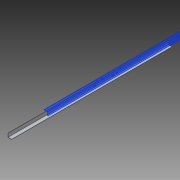
# Autodesk Inventor part: Shooter Back Support Bar
Saved by Autodesk Inventor 2014 SP1 (Build 180222100, 222)
## iProperties
Created: 2013-12-13
Part Number: Shooter Back Support Bar
Material: Aluminum 6061
Document SubType Name: Modeling
Designer: Moses
Mass: 45.3053 g
Surface Area: 433.276 cm^2
Volume: 16.7178 cm^3
Density: 2.71 g/cm^3
Appearance: Aluminum - Flat
Author: Moses
Autodesk Inventor part; units mm, degrees
ref_plane "YZ Plane" through (0, 0, 0) normal (1, 0, 0) x (0, 1, 0)
ref_plane "XZ Plane" through (0, 0, 0) normal (0, 1, 0) x (-1, 0, 0)
ref_plane "XY Plane" through (0, 0, 0) normal (0, 0, 1) x (1, 0, 0)
sketch "Sketch1" plane through (0, 0, 0) normal (0, 0, 1) x (1, 0, 0)
  line L0 (0, 0) -> (0, 15.875)
  line L1 (0, 15.875) -> (0.7937, 15.875)
  line L2 (0.7937, 15.875) -> (0.7938, 0.7937)
  line L3 (0.7938, 0.7937) -> (15.875, 0.7937)
  line L4 (15.875, 0.7937) -> (15.875, 0)
  line L5 (15.875, 0) -> (0, 0)
  dimension "d0" = 15.875
  dimension "d1" = 0.7937
  constraints: 12 end point, 3 horizontal, 3 vertical, 2 perpendicular
  measures "d0" distance of L0.start L0.end
  measures "d1" distance of L0.end L1.end
extrude "Extrusion1" add sketch "Sketch1" along normal blind 685.0063
sketch "Sketch2" plane through (0, 0, 0) normal (-1, 0, 0) x (0, 0, 1)
  line L0 (288.925, 278.403) -> (593.725, 278.403) construction
  arc A0 (593.725, 278.403) -> (593.725, 285.1594) centre (593.725, 281.7812) ccw construction
  line L1 (593.725, 285.1594) -> (288.925, 285.1594) construction
  arc A1 (288.925, 285.1594) -> (288.925, 278.403) centre (288.925, 281.7812) ccw construction
  circle A2 centre (657.225, 281.7812) radius 3.3782 construction
  circle A3 centre (625.475, 281.7812) radius 3.3782 construction
  line L2 (669.925, 294.4812) -> (669.925, 484.9812) construction
  line L3 (669.925, 484.9812) -> (200.025, 484.9812) construction
  line L4 (200.025, 484.9812) -> (200.025, 294.4812) construction
  line L5 (200.025, 294.4812) -> (669.925, 294.4812) construction
  line L6 (288.925, 151.403) -> (593.725, 151.403) construction
  arc A4 (593.725, 151.403) -> (593.725, 158.1594) centre (593.725, 154.7812) ccw construction
  line L7 (593.725, 158.1594) -> (288.925, 158.1594) construction
  arc A5 (288.925, 158.1594) -> (288.925, 151.403) centre (288.925, 154.7812) ccw construction
  ellipse E0 centre (657.225, 154.7796) end of major axis (653.8468, 154.7796) minor radius 3.3782 construction
  ellipse E1 centre (625.475, 154.7796) end of major axis (628.8532, 154.7796) minor radius 3.3782 construction
  line L8 (669.925, 269.0812) -> (200.025, 269.0812) construction
  line L9 (200.025, 269.0812) -> (200.025, 167.4812) construction
  line L10 (200.025, 167.4812) -> (669.925, 167.4812) construction
  line L11 (669.925, 167.4812) -> (669.925, 269.0812) construction
  line L12 (669.925, 15.0813) -> (669.925, 142.0812) construction
  line L13 (669.925, 142.0812) -> (200.025, 142.0812) construction
  line L14 (200.025, 142.0812) -> (200.025, 15.0813) construction
  line L15 (200.025, 15.0813) -> (669.925, 15.0813) construction
  circle A6 centre (676.275, 396.0812) radius 3.3782 construction
  circle A7 centre (193.675, 396.0812) radius 3.3782 construction
  circle A8 centre (676.275, 407.9875) radius 3.3782 construction
  circle A9 centre (193.675, 407.9875) radius 3.3782 construction
  circle A10 centre (676.275, 419.8937) radius 3.3782 construction
  circle A11 centre (193.675, 419.8937) radius 3.3782 construction
  circle A12 centre (676.275, 431.8) radius 3.3782 construction
  circle A13 centre (193.675, 431.8) radius 3.3782 construction
  circle A14 centre (676.275, 443.7062) radius 3.3782 construction
  circle A15 centre (193.675, 443.7062) radius 3.3782 construction
  circle A16 centre (676.275, 455.6125) radius 3.3782 construction
  circle A17 centre (193.675, 455.6125) radius 3.3782 construction
  circle A18 centre (676.275, 467.5187) radius 3.3782 construction
  circle A19 centre (193.675, 467.5187) radius 3.3782 construction
  circle A20 centre (676.275, 479.425) radius 3.3782 construction
  circle A21 centre (193.675, 479.425) radius 3.3782 construction
  circle A22 centre (676.275, 385.0141) radius 3.3782 construction
  circle A23 centre (193.675, 385.0141) radius 3.3782 construction
  circle A24 centre (676.275, 373.947) radius 3.3782 construction
  circle A25 centre (193.675, 373.947) radius 3.3782 construction
  circle A26 centre (676.275, 362.8798) radius 3.3782 construction
  circle A27 centre (193.675, 362.8798) radius 3.3782 construction
  circle A28 centre (676.275, 351.8127) radius 3.3782 construction
  circle A29 centre (193.675, 351.8127) radius 3.3782 construction
  circle A30 centre (676.275, 340.7455) radius 3.3782 construction
  circle A31 centre (193.675, 340.7455) radius 3.3782 construction
  circle A32 centre (676.275, 329.6784) radius 3.3782 construction
  circle A33 centre (193.675, 329.6784) radius 3.3782 construction
  circle A34 centre (676.275, 318.6112) radius 3.3782 construction
  circle A35 centre (193.675, 318.6112) radius 3.3782 construction
  circle A36 centre (676.275, 307.5441) radius 3.3782 construction
  circle A37 centre (193.675, 307.5441) radius 3.3782 construction
  circle A38 centre (676.275, 296.477) radius 3.3782 construction
  circle A39 centre (193.675, 296.477) radius 3.3782 construction
  circle A40 centre (676.275, 285.4098) radius 3.3782 construction
  circle A41 centre (193.675, 285.4098) radius 3.3782 construction
  circle A42 centre (676.275, 274.3427) radius 3.3782 construction
  circle A43 centre (193.675, 274.3427) radius 3.3782 construction
  circle A44 centre (676.275, 263.2755) radius 3.3782 construction
  circle A45 centre (193.675, 263.2755) radius 3.3782 construction
  circle A46 centre (676.275, 252.2084) radius 3.3782 construction
  circle A47 centre (193.675, 252.2084) radius 3.3782 construction
  circle A48 centre (676.275, 241.1412) radius 3.3782 construction
  circle A49 centre (193.675, 241.1412) radius 3.3782 construction
  circle A50 centre (676.275, 230.0741) radius 3.3782 construction
  circle A51 centre (193.675, 230.0741) radius 3.3782 construction
  circle A52 centre (676.275, 219.007) radius 3.3782 construction
  circle A53 centre (193.675, 219.007) radius 3.3782 construction
  circle A54 centre (676.275, 207.9398) radius 3.3782 construction
  circle A55 centre (193.675, 207.9398) radius 3.3782 construction
  circle A56 centre (676.275, 196.8727) radius 3.3782 construction
  circle A57 centre (193.675, 196.8727) radius 3.3782 construction
  circle A58 centre (676.275, 185.8055) radius 3.3782 construction
  circle A59 centre (193.675, 185.8055) radius 3.3782 construction
  circle A60 centre (676.275, 174.7384) radius 3.3782 construction
  circle A61 centre (193.675, 174.7384) radius 3.3782 construction
  circle A62 centre (676.275, 163.6712) radius 3.3782 construction
  circle A63 centre (193.675, 163.6712) radius 3.3782 construction
  circle A64 centre (676.275, 152.6041) radius 3.3782 construction
  circle A65 centre (193.675, 152.6041) radius 3.3782 construction
  circle A66 centre (676.275, 141.537) radius 3.3782 construction
  circle A67 centre (193.675, 141.537) radius 3.3782 construction
  circle A68 centre (676.275, 130.4698) radius 3.3782 construction
  circle A69 centre (193.675, 130.4698) radius 3.3782 construction
  circle A70 centre (676.275, 119.4027) radius 3.3782 construction
  circle A71 centre (193.675, 119.4027) radius 3.3782 construction
  circle A72 centre (676.275, 108.3355) radius 3.3782 construction
  circle A73 centre (193.675, 108.3355) radius 3.3782 construction
  circle A74 centre (676.275, 97.2684) radius 3.3782 construction
  circle A75 centre (193.675, 97.2684) radius 3.3782 construction
  circle A76 centre (676.275, 86.2012) radius 3.3782 construction
  circle A77 centre (193.675, 86.2012) radius 3.3782 construction
  circle A78 centre (676.275, 75.1341) radius 3.3782 construction
  circle A79 centre (193.675, 75.1341) radius 3.3782 construction
  circle A80 centre (676.275, 64.067) radius 3.3782 construction
  circle A81 centre (193.675, 64.067) radius 3.3782 construction
  circle A82 centre (676.275, 52.9998) radius 3.3782 construction
  circle A83 centre (193.675, 52.9998) radius 3.3782 construction
  circle A84 centre (676.275, 41.9327) radius 3.3782 construction
  circle A85 centre (193.675, 41.9327) radius 3.3782 construction
  circle A86 centre (676.275, 30.8655) radius 3.3782 construction
  circle A87 centre (193.675, 30.8655) radius 3.3782 construction
  circle A88 centre (676.275, 19.7984) radius 3.3782 construction
  circle A89 centre (193.675, 19.7984) radius 3.3782 construction
  circle A90 centre (676.275, 491.3312) radius 3.3782 construction
  circle A91 centre (666.426, 491.3312) radius 3.3782 construction
  circle A92 centre (656.577, 491.3312) radius 3.3782 construction
  circle A93 centre (646.7281, 491.3312) radius 3.3782 construction
  circle A94 centre (636.8791, 491.3312) radius 3.3782 construction
  circle A95 centre (627.0301, 491.3312) radius 3.3782 construction
  circle A96 centre (617.1811, 491.3312) radius 3.3782 construction
  circle A97 centre (607.3321, 491.3312) radius 3.3782 construction
  circle A98 centre (597.4832, 491.3312) radius 3.3782 construction
  circle A99 centre (587.6342, 491.3312) radius 3.3782 construction
  circle A100 centre (577.7852, 491.3312) radius 3.3782 construction
  circle A101 centre (567.9362, 491.3312) radius 3.3782 construction
  circle A102 centre (558.0872, 491.3312) radius 3.3782 construction
  circle A103 centre (548.2383, 491.3312) radius 3.3782 construction
  circle A104 centre (538.3893, 491.3312) radius 3.3782 construction
  circle A105 centre (528.5403, 491.3312) radius 3.3782 construction
  circle A106 centre (518.6913, 491.3312) radius 3.3782 construction
  circle A107 centre (508.8423, 491.3312) radius 3.3782 construction
  circle A108 centre (498.9934, 491.3312) radius 3.3782 construction
  circle A109 centre (489.1444, 491.3312) radius 3.3782 construction
  circle A110 centre (479.2954, 491.3312) radius 3.3782 construction
  circle A111 centre (469.4464, 491.3312) radius 3.3782 construction
  circle A112 centre (459.5974, 491.3312) radius 3.3782 construction
  circle A113 centre (449.7485, 491.3312) radius 3.3782 construction
  circle A114 centre (439.8995, 491.3312) radius 3.3782 construction
  circle A115 centre (430.0505, 491.3312) radius 3.3782 construction
  circle A116 centre (420.2015, 491.3312) radius 3.3782 construction
  circle A117 centre (410.3526, 491.3312) radius 3.3782 construction
  circle A118 centre (400.5036, 491.3312) radius 3.3782 construction
  circle A119 centre (390.6546, 491.3312) radius 3.3782 construction
  circle A120 centre (380.8056, 491.3312) radius 3.3782 construction
  circle A121 centre (370.9566, 491.3312) radius 3.3782 construction
  circle A122 centre (361.1077, 491.3312) radius 3.3782 construction
  circle A123 centre (351.2587, 491.3312) radius 3.3782 construction
  circle A124 centre (341.4097, 491.3312) radius 3.3782 construction
  circle A125 centre (331.5607, 491.3312) radius 3.3782 construction
  circle A126 centre (321.7117, 491.3312) radius 3.3782 construction
  circle A127 centre (311.8628, 491.3312) radius 3.3782 construction
  circle A128 centre (302.0138, 491.3312) radius 3.3782 construction
  circle A129 centre (292.1648, 491.3312) radius 3.3782 construction
  circle A130 centre (282.3158, 491.3312) radius 3.3782 construction
  circle A131 centre (272.4668, 491.3312) radius 3.3782 construction
  circle A132 centre (262.6179, 491.3312) radius 3.3782 construction
  circle A133 centre (252.7689, 491.3312) radius 3.3782 construction
  circle A134 centre (242.9199, 491.3312) radius 3.3782 construction
  circle A135 centre (233.0709, 491.3312) radius 3.3782 construction
  circle A136 centre (223.2219, 491.3312) radius 3.3782 construction
  circle A137 centre (213.373, 491.3312) radius 3.3782 construction
  circle A138 centre (203.524, 491.3312) radius 3.3782 construction
  circle A139 centre (193.675, 491.3312) radius 3.3782 construction
  circle A140 centre (676.275, 8.7313) radius 3.3782 projected
  circle A141 centre (666.426, 8.7313) radius 3.3782 construction
  circle A142 centre (656.577, 8.7313) radius 3.3782 construction
  circle A143 centre (646.7281, 8.7313) radius 3.3782 construction
  circle A144 centre (636.8791, 8.7313) radius 3.3782 construction
  circle A145 centre (627.0301, 8.7313) radius 3.3782 construction
  circle A146 centre (617.1811, 8.7313) radius 3.3782 construction
  circle A147 centre (607.3321, 8.7313) radius 3.3782 construction
  circle A148 centre (597.4832, 8.7313) radius 3.3782 construction
  circle A149 centre (587.6342, 8.7313) radius 3.3782 construction
  circle A150 centre (577.7852, 8.7313) radius 3.3782 construction
  circle A151 centre (567.9362, 8.7313) radius 3.3782 construction
  circle A152 centre (558.0872, 8.7313) radius 3.3782 construction
  circle A153 centre (548.2383, 8.7313) radius 3.3782 construction
  circle A154 centre (538.3893, 8.7313) radius 3.3782 construction
  circle A155 centre (528.5403, 8.7313) radius 3.3782 construction
  circle A156 centre (518.6913, 8.7313) radius 3.3782 construction
  circle A157 centre (508.8423, 8.7313) radius 3.3782 construction
  circle A158 centre (498.9934, 8.7313) radius 3.3782 construction
  circle A159 centre (489.1444, 8.7313) radius 3.3782 construction
  circle A160 centre (479.2954, 8.7313) radius 3.3782 construction
  circle A161 centre (469.4464, 8.7313) radius 3.3782 construction
  circle A162 centre (459.5974, 8.7313) radius 3.3782 construction
  circle A163 centre (449.7485, 8.7313) radius 3.3782 construction
  circle A164 centre (439.8995, 8.7313) radius 3.3782 construction
  circle A165 centre (430.0505, 8.7313) radius 3.3782 construction
  circle A166 centre (420.2015, 8.7313) radius 3.3782 construction
  circle A167 centre (410.3526, 8.7313) radius 3.3782 construction
  circle A168 centre (400.5036, 8.7313) radius 3.3782 construction
  circle A169 centre (390.6546, 8.7313) radius 3.3782 construction
  circle A170 centre (380.8056, 8.7313) radius 3.3782 construction
  circle A171 centre (370.9566, 8.7313) radius 3.3782 construction
  circle A172 centre (361.1077, 8.7313) radius 3.3782 construction
  circle A173 centre (351.2587, 8.7313) radius 3.3782 construction
  circle A174 centre (341.4097, 8.7313) radius 3.3782 construction
  circle A175 centre (331.5607, 8.7313) radius 3.3782 construction
  circle A176 centre (321.7117, 8.7313) radius 3.3782 construction
  circle A177 centre (311.8628, 8.7313) radius 3.3782 construction
  circle A178 centre (302.0138, 8.7313) radius 3.3782 construction
  circle A179 centre (272.4668, 8.7313) radius 3.3782 construction
  circle A180 centre (262.6179, 8.7313) radius 3.3782 construction
  circle A181 centre (252.7689, 8.7313) radius 3.3782 construction
  circle A182 centre (242.9199, 8.7313) radius 3.3782 construction
  circle A183 centre (233.0709, 8.7313) radius 3.3782 construction
  circle A184 centre (223.2219, 8.7313) radius 3.3782 construction
  circle A185 centre (213.373, 8.7313) radius 3.3782 projected
  circle A186 centre (203.524, 8.7313) radius 3.3782 construction
  circle A187 centre (193.675, 8.7313) radius 3.3782 projected
  line L16 (682.625, 2.3813) -> (187.325, 2.3813) construction
  line L17 (187.325, 2.3813) -> (187.325, 497.6812) construction
  line L18 (187.325, 497.6812) -> (682.625, 497.6812) construction
  line L19 (682.625, 497.6812) -> (682.625, 2.3813) construction
  circle A188 centre (477.7908, 396.0812) radius 3.3782 construction
  circle A189 centre (398.6756, 286.3307) radius 3.3782 construction
  circle A190 centre (422.4733, 262.533) radius 3.3782 construction
  circle A191 centre (444.1358, 396.0812) radius 3.3782 construction
  line L20 (418.0849, 248.9608) -> (558.1878, 108.8579) construction
  arc A192 (558.1878, 108.8579) -> (576.1483, 126.8184) centre (288.925, 396.0812) ccw construction
  line L21 (576.1483, 126.8184) -> (323.3053, 379.6615) construction
  arc A193 (323.3053, 379.6615) -> (326.4921, 389.7312) centre (288.925, 396.0812) ccw construction
  line L22 (326.4921, 389.7312) -> (682.5738, 389.7312) construction
  arc A194 (682.5738, 389.7312) -> (682.625, 396.0812) centre (288.925, 396.0812) ccw construction
  line L23 (682.625, 396.0812) -> (682.625, 402.4312) construction
  line L24 (682.625, 402.4312) -> (326.4921, 402.4312) construction
  arc A195 (326.4921, 402.4312) -> (282.575, 358.5141) centre (288.925, 396.0812) ccw construction
  line L25 (282.575, 358.5141) -> (282.575, 296.4095) construction
  arc A196 (295.275, 281.641) -> (282.575, 296.4095) centre (178.435, 194.011) ccw construction
  line L26 (295.275, 281.641) -> (360.9975, 194.011) construction
  line L27 (360.9975, 194.011) -> (295.275, 106.381) construction
  arc A197 (282.575, 91.6124) -> (295.275, 106.381) centre (178.435, 194.011) ccw construction
  line L28 (282.575, 91.6124) -> (282.575, 2.3812) construction
  line L29 (282.575, 2.3812) -> (288.925, 2.3812) construction
  arc A198 (288.925, 2.3812) -> (295.275, 2.4325) centre (288.925, 396.0812) ccw construction
  line L30 (295.275, 2.4325) -> (295.275, 85.2143) construction
  line L31 (295.275, 85.2143) -> (418.0849, 248.9608) construction
  circle A199 centre (288.925, 8.7312) radius 3.3782 projected
  circle A200 centre (288.925, 59.5312) radius 3.3782 construction
  line L32 (409.0135, 258.0323) -> (368.935, 204.5943) construction
  line L33 (368.935, 204.5943) -> (295.275, 302.8076) construction
  line L34 (295.275, 302.8076) -> (295.275, 358.5141) construction
  arc A201 (295.275, 358.5141) -> (305.3447, 361.701) centre (288.925, 396.0812) ccw construction
  line L35 (305.3447, 361.701) -> (409.0135, 258.0323) construction
  circle A202 centre (288.925, 396.0812) radius 9.5 construction
  circle A203 centre (559.1526, 118.5617) radius 3.3782 construction
  circle A204 centre (566.4445, 125.8537) radius 3.3782 construction
  circle A205 centre (523.2315, 154.4828) radius 3.3782 construction
  circle A206 centre (530.5235, 161.7747) radius 3.3782 construction
  circle A207 centre (676.275, 396.0812) radius 3.3782 construction
  circle A208 centre (625.475, 396.0812) radius 3.3782 construction
  circle A209 centre (428.625, 396.0812) radius 3.3782 construction
  circle A210 centre (568.325, 396.0812) radius 3.3782 construction
  circle A211 centre (383.1156, 292.9104) radius 3.3782 construction
  circle A212 centre (392.0958, 301.8907) radius 3.3782 construction
  circle A213 centre (481.9495, 194.0765) radius 3.3782 construction
  circle A214 centre (490.9297, 203.0568) radius 3.3782 construction
  arc A215 (291.0239, 5.5515) -> (291.0239, 11.911) centre (292.1648, 8.7313) ccw projected
  arc A216 (285.3856, 10.1415) -> (285.3856, 7.321) centre (282.3158, 8.7313) ccw projected
  arc A217 (291.0239, 11.911) -> (285.3856, 10.1415) centre (288.925, 8.7312) ccw projected
  arc A218 (285.3856, 7.321) -> (291.0239, 5.5515) centre (288.925, 8.7312) ccw projected
  constraints: 2 other
extrude "Extrusion2" cut sketch "Sketch2" against normal through all contours A140 | A185 | A187 | A199
body "Solid1"
